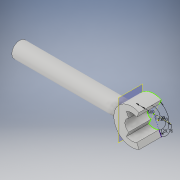
# Autodesk Inventor part: golf2
Saved by Autodesk Inventor 2018.3 (Build 223284000, 284)
## iProperties
Created: 2019-05-03
Part Number: golf2
Material: Generic
Document SubType Name: Modeling
Designer: F8PLTW
Density: 1 g/cm^3
Appearance: Default
Author: F8PLTW
Autodesk Inventor part; units mm, degrees
ref_plane "YZ Plane" through (0, 0, 0) normal (1, 0, 0) x (0, 1, 0)
ref_plane "XZ Plane" through (0, 0, 0) normal (0, 1, 0) x (-1, 0, 0)
ref_plane "XY Plane" through (0, 0, 0) normal (0, 0, 1) x (1, 0, 0)
sketch "Sketch1" plane through (0, 0, 0) normal (0, 0, 1) x (1, 0, 0)
  arc A0 (0.5408, 16.1042) -> (0.5408, -9.1933) centre (-5.3897, 3.4555) ccw
  arc A1 (3.2365, 21.8536) -> (3.2365, -14.9427) centre (-5.3897, 3.4555) ccw
  arc A2 (-8.6245, 10.3548) -> (-12.2365, 0.111) centre (-5.3897, 3.4555) ccw
  line L0 (-11.3201, 16.1042) -> (-8.6245, 10.3548)
  line L1 (-5.3897, 3.4555) -> (3.2365, 21.8536) construction
  line L2 (-5.3897, 3.4555) -> (3.2365, -14.9427) construction
  line L3 (-5.3897, 3.4555) -> (14.9303, 3.4555) construction
  line L4 (-5.3897, 3.4555) -> (-14.0158, -14.9427) construction
  line L5 (-5.3897, 3.4555) -> (-14.0158, 21.8536) construction
  arc A3 (-8.6245, 10.3548) -> (-8.6245, -3.4438) centre (-5.3897, 3.4555) ccw
  line L6 (-8.6245, -3.4438) -> (-11.3201, -9.1933)
  line L7 (0.5408, 16.1042) -> (3.2365, 21.8536)
  line L8 (0.5408, -9.1933) -> (3.2365, -14.9427)
  line L9 (-19.3597, 3.4555) -> (-19.3597, -7.0739) construction
  point P0 (0, 0)
  dimension "d0" = 27.94
  dimension "d1" = 40.64
  dimension "d2" = 15.24
  dimension "d4" = 129.76
  constraints: 20 end point, 14 point on circle, 5 point on line, 4 centre point, 3 coincident, 3 collinear, 1 horizontal, 1 tangent, 1 vertical, 2 other
  measures "d0" diameter of A0
  measures "d1" diameter of A1
  measures "d2" diameter of A2
  measures "d4" angle of L2 L1
extrude "Extrusion1" add sketch "Sketch1" along normal blind 25.4
ref_plane "Work Plane1" through (-19.3597, 3.4555, 0) normal (-1, 0, 0) x (0, -1, 0)
sketch "Sketch2" plane through (-19.3597, 3.4555, 0) normal (-1, 0, 0) x (0, -1, 0)
  line L0 (-20.32, 0) -> (-20.32, 25.4) projected
  line L1 (20.32, 25.4) -> (-20.32, 25.4) projected
  line L2 (-20.32, 0) -> (20.32, 25.4)
  line L3 (-20.32, 25.4) -> (20.32, 0)
  line L4 (20.32, 0) -> (20.32, 25.4) projected
  circle A0 centre (0, 12.7) radius 8.89
  point P0 (3.4555, 0)
  point P1 (-18.3981, 25.4)
  point P2 (18.3981, 25.4)
  dimension "d7" = 17.78
  constraints: 4 end point, 2 point on line, 1 centre point, 1 midpoint
  measures "d7" diameter of A0
extrude "Extrusion2" add sketch "Sketch2" along normal blind 127 contours A0 L3 L2 | L2 L3 A0 | A0 L2 L3 | L2 A0 L3
body "Solid1"
